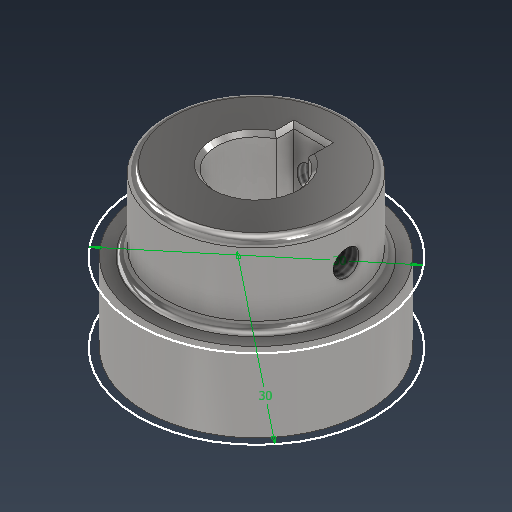
# Autodesk Inventor part: gear_khk_SUS1-28J10
Saved by Autodesk Inventor 2021 (Build 250183000, 183)
## iProperties
Created: 2021-06-22
Part Number: gear_khk_SUS1-28J10
Material: Steel, High Strength, Low Alloy
Document SubType Name: Modeling
Designer: Watchdog
Density: 7.85 g/cm^3
Appearance: Steel - Polished
Author: Watchdog
Autodesk Inventor part; units mm, degrees
ref_plane "XZ Plane" through (0, 0, 0) normal (0, 1, 0) x (-1, 0, 0)
sketch "Sketch1" plane through (0, 0, 0) normal (0, 1, 0) x (-1, 0, 0)
  circle A0 centre (0, 0) radius 5
  circle A1 centre (0, 0) radius 14
  dimension "d0" = 10
  dimension "d1" = 28
  constraints: 2 centre point, 2 coincident
  measures "d0" diameter of A0
  measures "d1" diameter of A1
extrude "Extrusion1" add sketch "Sketch1" along normal blind 10
sketch "Sketch2" plane through (0, 10, 0) normal (0, 1, 0) x (1, 0, 0)
  circle A0 centre (0, 0) radius 11.5
  circle A1 centre (0, 0) radius 5 projected
  dimension "d4" = 23
  constraints: 1 centre point
  measures "d4" diameter of A0
extrude "Extrusion2" add sketch "Sketch2" along normal blind 10
fillet "Fillet1" radius 1 1 edges at (-11.5, 10, 0)
ref_plane "Work Plane1" through (11.5, 10, 0) normal (1, 0, 0) x (0, 1, 0)
fillet "Fillet2" radius 1 1 edges at (-11.5, 20, 0)
ref_plane "Work Plane2" through (0, 10, -11.5) normal (0, 0, 1) x (1, 0, 0)
sketch "Sketch4" plane through (0, 10, -11.5) normal (0, 0, 1) x (1, 0, 0)
  line L0 (-10.5, 10) -> (10.5, 10) projected
  point P0 (0, -10)
  point P1 (0, 5)
  dimension "d21" = 5
  dimension "d22" = 0
  measures "d21" distance from line of L0 point (0, 5)
  measures "d22" horizontal distance of point (0, -10) point (0, 5)
sketch "Sketch3" plane through (11.5, 10, 0) normal (1, 0, 0) x (0, 1, 0)
  line L0 (10, -11.5) -> (10, 11.5) projected
  point P0 (-10, 0)
  point P1 (5, 0)
  dimension "d8" = 5
  dimension "d9" = 0
  measures "d8" distance from line of L0 point (5, 0)
  measures "d9" vertical distance of point (-10, 0) point (5, 0)
hole "Hole1" at (11.5, 15, 0) direction (-1, 0, 0) diameter 3.242 end up to face face through (0, 0, 0) facing (0, 1, 0) round with radius 5 far side no thread size "M4x0.7" class "6H" standard "ISO Metric profile"
hole "Hole2" at (0, 15, -11.5) direction (0, 0, 1) diameter 3.242 end up to face face through (0, 0, 0) facing (0, 1, 0) round with radius 5 far side no thread size "M4x0.7" class "6H" standard "ISO Metric profile"
sketch "Sketch5" plane through (0, 20, 0) normal (0, 1, 0) x (1, 0, 0)
  line L0 (-2, 4.5826) -> (2, 4.5826)
  line L1 (2, 4.5826) -> (2, 6.8)
  line L2 (2, 6.8) -> (-2, 6.8)
  line L3 (-2, 6.8) -> (-2, 4.5826)
  circle A0 centre (0, 0) radius 5 projected
  dimension "d30" = 4
  dimension "d31" = 6.8
  constraints: 8 end point, 2 parallel, 2 point on circle, 1 horizontal, 1 perpendicular
  measures "d30" distance between parallel lines of L1 L3
  measures "d31" distance from line of L2 point (0, 0)
extrude "Extrusion3" cut sketch "Sketch5" against normal through all contours A0 L0 | L3 L2 L1 A0 picked at (0.3405, 4.6866)
chamfer "Chamfer2" distance 0.5 angle 45 8 edges at (-2, 20, -5.6913) (0, 20, -6.8) (2, 20, -5.6913) (0, 20, 5) (0, 0, -6.8) (-2, 0, -5.6913) (2, 0, -5.6913) (0, 0, 5)
sketch "Sketch6" plane through (0, 0, 0) normal (0, -1, 0) x (1, 0, 0)
  circle A0 centre (0, 0) radius 15
  dimension "d37" = 30
  constraints: 1 centre point, 1 coincident
  measures "d37" diameter of A0
sketch "Sketch7" plane through (0, 10, 0) normal (0, 1, 0) x (1, 0, 0)
  circle A0 centre (0, 0) radius 15
  dimension "d38" = 30
  constraints: 1 centre point, 1 coincident
  measures "d38" diameter of A0
body "Solid1"
